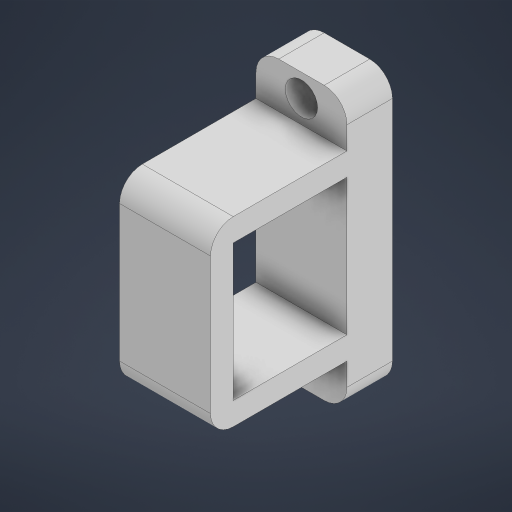
# Autodesk Inventor part: Latch_For_Climb_And_Drone
Saved by Autodesk Inventor 2023 (Build 270158000, 158)
## iProperties
Created: 2024-02-26
Part Number: Latch_For_Climb_And_Drone
Material: Generic
Document SubType Name: Modeling
Designer: kelle
Density: 1 g/cm^3
Appearance: Default
Author: kelle
Autodesk Inventor part; units mm, degrees
ref_plane "YZ Plane" through (0, 0, 0) normal (1, 0, 0) x (0, 1, 0)
ref_plane "XZ Plane" through (0, 0, 0) normal (0, 1, 0) x (-1, 0, 0)
ref_plane "XY Plane" through (0, 0, 0) normal (0, 0, 1) x (1, 0, 0)
sketch "Sketch1" plane through (0, 0, 0) normal (0, 0, 1) x (1, 0, 0)
  line L0 (6.35, -12.7) -> (-6.35, -12.7)
  line L1 (-6.35, -12.7) -> (-6.35, 12.7)
  line L2 (-6.35, 12.7) -> (6.35, 12.7)
  line L3 (6.35, 12.7) -> (6.35, -12.7)
  line L4 (6.35, -12.7) -> (-6.35, 12.7) construction
  line L5 (-6.35, -12.7) -> (6.35, 12.7) construction
  line L6 (-6.35, 12.7) -> (6.35, 12.7)
  line L7 (6.35, 12.7) -> (6.35, 19.05)
  line L8 (6.35, 19.05) -> (-6.35, 19.05)
  line L9 (-6.35, 19.05) -> (-6.35, 12.7)
  line L10 (-6.35, -12.7) -> (6.35, -12.7)
  line L11 (6.35, -12.7) -> (6.35, -19.05)
  line L12 (6.35, -19.05) -> (-6.35, -19.05)
  line L13 (-6.35, -19.05) -> (-6.35, -12.7)
  circle A0 centre (0, 15.875) radius 2.25
  circle A1 centre (0, -15.875) radius 2.25
  point P0 (0, 0)
  dimension "d0" = 12.7
  dimension "d1" = 25.4
  dimension "d2" = 6.35
  dimension "d3" = 6.35
  dimension "d4" = 4.5
  dimension "d5" = 4.5
  constraints: 28 end point, 6 parallel, 3 horizontal, 3 perpendicular, 2 centre point, 2 midpoint
  measures "d0" distance of L1.end L2.end
  measures "d1" distance of L0.end L1.end
  measures "d2" distance of L7.end L6.end
  measures "d3" distance of L10.end L11.end
  measures "d4" diameter of A0
  measures "d5" diameter of A1
extrude "Extrusion1" add sketch "Sketch1" along normal blind 6.35 contours L11 L12 L13 L0 | L2 L9 L8 L7
extrude "Extrusion2" add sketch "Sketch1" along normal blind 25.4 contours L0 L1 L2 L3
sketch "Sketch2" plane through (6.35, -19.05, 0) normal (1, 0, 0) x (0, 0, -1)
  line L0 (0, 0) -> (0, 38.1) projected
  line L1 (0, 38.1) -> (-6.35, 38.1) projected
  line L2 (-6.35, 31.75) -> (-6.35, 38.1) projected
  line L3 (-6.35, 31.75) -> (-25.4, 31.75) projected
  line L4 (-25.4, 6.35) -> (-25.4, 31.75) projected
  line L5 (-6.35, 6.35) -> (-25.4, 6.35) projected
  line L6 (-6.35, 0) -> (-6.35, 6.35) projected
  line L7 (0, 0) -> (-6.35, 0) projected
  line L8 (-6.35, 38.1) -> (-6.35, 31.75) projected
  line L9 (-6.35, 6.35) -> (-6.35, 0) projected
  line L10 (-6.35, 31.75) -> (-6.35, 6.35)
  line L11 (-6.35, 28.575) -> (-22.225, 28.575)
  line L12 (-22.225, 28.575) -> (-22.225, 9.525)
  line L13 (-22.225, 9.525) -> (-6.35, 9.525)
  point P0 (0, 19.05)
  dimension "d10" = 3.175
  constraints: 8 end point, 2 other
  measures "d10" distance between parallel lines of L3 L11
extrude "Extrusion3" cut sketch "Sketch2" against normal through all contours L13 L12 L11 L10
fillet "Fillet1" radius 3.175 6 edges at (-6.35, 19.05, 3.175) (6.35, 19.05, 3.175) (0, 12.7, 25.4) (0, -12.7, 25.4) (6.35, -19.05, 3.175) (-6.35, -19.05, 3.175)
body "Solid1"
